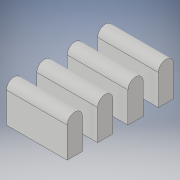
# Autodesk Inventor part: cup mount
Saved by Autodesk Inventor 2019.3 (Build 233278000, 278)
## iProperties
Created: 2019-07-22
Part Number: cup mount
Material: Generic
Document SubType Name: Modeling
Designer: Frienddo
Density: 1 g/cm^3
Appearance: Default
Author: Frienddo
Autodesk Inventor part; units mm, degrees
ref_plane "YZ Plane" through (0, 0, 0) normal (1, 0, 0) x (0, 1, 0)
ref_plane "XZ Plane" through (0, 0, 0) normal (0, 1, 0) x (-1, 0, 0)
ref_plane "XY Plane" through (0, 0, 0) normal (0, 0, 1) x (1, 0, 0)
sketch "Sketch1" plane through (0, 0, 0) normal (1, 0, 0) x (0, 1, 0)
  line L0 (0, 12.5) -> (10, 12.5)
  line L1 (10, 12.5) -> (10, 17.5)
  line L2 (10, 17.5) -> (0, 17.5)
  line L3 (0, 17.5) -> (0, 12.5)
  arc A0 (10, 12.5) -> (10, 17.5) centre (10, 15) ccw
  line L4 (0, 2.5) -> (10, 2.5)
  line L5 (10, 2.5) -> (10, 7.5)
  line L6 (10, 7.5) -> (0, 7.5)
  line L7 (0, 7.5) -> (0, 2.5)
  arc A1 (10, 2.5) -> (10, 7.5) centre (10, 5) ccw
  line L8 (0, -7.5) -> (10, -7.5)
  line L9 (10, -7.5) -> (10, -2.5)
  line L10 (10, -2.5) -> (0, -2.5)
  line L11 (0, -2.5) -> (0, -7.5)
  arc A2 (10, -7.5) -> (10, -2.5) centre (10, -5) ccw
  line L12 (0, -17.5) -> (10, -17.5)
  line L13 (10, -17.5) -> (10, -12.5)
  line L14 (10, -12.5) -> (0, -12.5)
  line L15 (0, -12.5) -> (0, -17.5)
  arc A3 (10, -17.5) -> (10, -12.5) centre (10, -15) ccw
  line L16 (0, 2.5) -> (0, -2.5) construction
  point P0 (0, 0)
  point P1 (0, 0)
  dimension "d0" = 10
  dimension "d1" = 5
  dimension "d4" = 10
  constraints: 34 end point, 8 point on circle, 4 centre point, 2 collinear, 2 midpoint, 2 parallel, 2 perpendicular, 2 point on line, 1 coincident, 1 horizontal, 1 vertical, 29 other
  measures "d0" distance of L2.end L1.end
  measures "d1" distance of L0.end L1.end
  measures "d4" distance of L0.start L4.start
extrude "Extrusion1" add sketch "Sketch1" along normal mid plane 20
body "Solid1"
